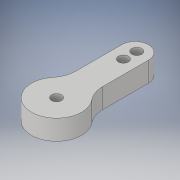
# Autodesk Inventor part: orczyk_powerHD
Saved by Autodesk Inventor 2019 (Build 230136000, 136)
## iProperties
Created: 2021-11-19
Part Number: orczyk_powerHD
Material: Generic
Document SubType Name: Modeling
Designer: Pokick
Density: 1 g/cm^3
Appearance: Default
Author: Pokick
Autodesk Inventor part; units mm, degrees
ref_plane "YZ Plane" through (0, 0, 0) normal (1, 0, 0) x (0, 1, 0)
ref_plane "XZ Plane" through (0, 0, 0) normal (0, 1, 0) x (-1, 0, 0)
ref_plane "XY Plane" through (0, 0, 0) normal (0, 0, 1) x (1, 0, 0)
sketch "Sketch1" plane through (0, 0, 0) normal (0, 1, 0) x (-1, 0, 0)
  circle A0 centre (0, 0) radius 7.5 construction
  line L0 (0, 7.5) -> (0, -27.5) construction
  line L1 (0, -27.5) -> (0, -23.5) construction
  circle A1 centre (0, -23.5) radius 4 construction
  circle A2 centre (0, 0) radius 7.5
  circle A3 centre (0, -23.5) radius 4
  line L2 (-4, -23.5) -> (-4, -6.3443)
  line L3 (4, -23.5) -> (4, -6.3443)
  dimension "d0" = 15
  dimension "d1" = 35
  dimension "d2" = 0
  dimension "d3" = 4
  constraints: 8 end point, 5 point on circle, 4 coincident, 4 vertical, 2 centre point, 2 tangent, 2 vertical alignment, 1 point on line, 5 other
  measures "d1" distance of L0.start L0.end
  measures "d2" distance from line of point (0, 0) L0
  measures "d3" distance of L0.end L1.end
extrude "Extrusion1" add sketch "Sketch1" along normal blind 6
fillet "Fillet1" radius 8 2 edges at (-4, 3, -6.3443) (4, 3, -6.3443)
sketch "Sketch2" plane through (0, 0, 0) normal (0, -1, 0) x (1, 0, 0)
  line L0 (0, 0) -> (0, -27.5) construction
  arc A0 (-4, -23.5) -> (4, -23.5) centre (0, -23.5) ccw projected
  line L1 (0, -27.5) -> (0, -24) construction
  circle A1 centre (0, -24) radius 1.5
  line L2 (0, -24) -> (0, -20) construction
  circle A2 centre (0, -20) radius 1.5
  circle A3 centre (0, 0) radius 1.5
  dimension "d8" = 3.5
  dimension "d9" = 3
  dimension "d10" = 4
  dimension "d11" = 3
  dimension "d12" = 3
  constraints: 6 end point, 3 centre point, 3 coincident, 2 point on line, 1 point on circle, 1 vertical
  measures "d8" distance of L0.end L1.end
  measures "d9" diameter of A1
  measures "d10" distance of L2.start L2.end
  measures "d11" diameter of A2
  measures "d12" diameter of A3
extrude "Extrusion2" cut sketch "Sketch2" against normal blind 6
sketch "Sketch3" plane through (0, 0, 0) normal (0, -1, 0) x (1, 0, 0)
  circle A0 centre (0, 0) radius 2.8
  dimension "d15" = 5.6
  constraints: 1 centre point, 1 coincident
  measures "d15" diameter of A0
extrude "Extrusion3" cut sketch "Sketch3" against normal blind 3
body "Solid1"
